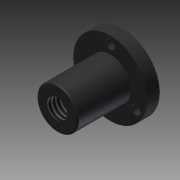
# Autodesk Inventor part: LeadScrewNut
Saved by Autodesk Inventor 2011 (Build 150239000, 239)
## iProperties
Company: FirstCadLibrary
Shininess: 64.0
Length Units: 11272
Angle Units: 11279
Time Units: 11290
Mass Units: 11283
Length Display Precision: 3
Angle Display Precision: 2
Compacted: True
Part Number: LeadScrewNut
Document SubType Name: Modeling
Created: 2007-01-12
Material: ABS Plastic
Designer: Ed Sparks
Catalog Web Link: www.kerkmotion.com
Vendor: Kerk Motion
Description: Lead Screw Nut
Density: 1 g/cm^3
Density: 0.0
Volumn: 0.0
Area: 0.0
PropertySet Name: Model Information
Control State: 0
Master: False
Checked Out: False
Author: Ed Sparks
Autodesk Inventor part; units mm, degrees
ref_plane "YZ Plane" through (0, 0, 0) normal (1, 0, 0) x (0, 1, 0)
ref_plane "XZ Plane" through (0, 0, 0) normal (0, 1, 0) x (-1, 0, 0)
ref_plane "XY Plane" through (0, 0, 0) normal (0, 0, 1) x (1, 0, 0)
sketch "Sketch1" plane through (0, 0, 0) normal (0, 0, 1) x (1, 0, 0)
  circle A0 centre (0, 0) radius 8.001
  dimension "d0" = 16.002
  constraints: 2 coincident, 1 centre point, 2 other
  measures "d0" diameter of A0
extrude "Extrusion1" add sketch "Sketch1" along normal mid plane 20.574
sketch "Sketch2" plane through (0, 0, 10.287) normal (0, 0, 1) x (1, 0, 0)
  circle A0 centre (0, 0) radius 8.001 projected
  circle A1 centre (0, 0) radius 14.351
  dimension "d29" = 28.702
  constraints: 2 coincident, 1 centre point, 1 other
  measures "d29" diameter of A1
extrude "Extrusion2" add sketch "Sketch2" along normal blind 4.826 contours A0 | A1
sketch "Sketch4" plane through (0, 0, -10.287) normal (0, 0, -1) x (-1, 0, 0)
  circle A0 centre (0, 0) radius 8.001 projected
  constraints: 1 coincident
hole "Hole2" at (0, 0, -10.287) direction (0, 0, 1) diameter 7.7978 end through all thread size "3/8-16 UNC" class "2B" standard "ANSI Unified Screw Threads"
chamfer "Chamfer1" distance 0.381 angle 45 1 edges at (-8.001, 0, -10.287)
sketch "Sketch6" plane through (0, 0, 15.113) normal (0, 0, 1) x (1, 0, 0)
  circle A0 centre (0, 0) radius 14.351 projected
  circle A1 centre (0, 0) radius 11.4134 construction
  point P0 (0, 11.4134)
  constraints: 1 coincident, 1 vertical alignment, 2 other
hole "Hole3" at (0, 11.4134, 15.113) direction (0, 0, -1) diameter 3.556 end through all
pattern_circular "Circular Pattern1" count 3 over 360 about axis through (0, 0, 10.287) along (0, 0, 1) of "Hole3"
body "Solid1"
